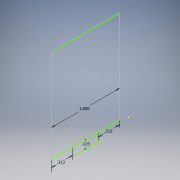
# Autodesk Inventor part: Part16
Saved by Autodesk Inventor 2018 (Build 220112000, 112)
## iProperties
Created: 2018-05-23
Part Number: Part16
Material: Generic
Document SubType Name: Modeling
Designer: lenovo
Density: 1 g/cm^3
Appearance: Default
Author: lenovo
Autodesk Inventor part; units mm, degrees
ref_plane "YZ Plane" through (0, 0, 0) normal (1, 0, 0) x (0, 1, 0)
ref_plane "XZ Plane" through (0, 0, 0) normal (0, 1, 0) x (-1, 0, 0)
ref_plane "XY Plane" through (0, 0, 0) normal (0, 0, 1) x (1, 0, 0)
sketch "Sketch1" plane through (0, 0, 0) normal (1, 0, 0) x (0, 1, 0)
  line L0 (35.589, 28.7672) -> (-47.596, 28.7672)
  line L1 (-47.596, 28.7672) -> (-47.596, 3.3672)
  line L2 (-47.596, 3.3672) -> (35.589, 3.3672)
  line L3 (35.589, 3.3672) -> (35.589, 28.7672)
  line L4 (-47.596, 20.8297) -> (-50.771, 20.8297)
  line L5 (-50.771, 20.8297) -> (-50.771, 11.3047)
  line L6 (-50.771, 11.3047) -> (-47.596, 11.3047)
  line L7 (-47.596, 11.3047) -> (-47.596, 20.8297)
  line L8 (-39.6585, 28.7672) -> (-30.1335, 28.7672)
  line L9 (-30.1335, 28.7672) -> (-30.1335, 25.5922)
  line L10 (-30.1335, 25.5922) -> (-39.6585, 25.5922)
  line L11 (-39.6585, 25.5922) -> (-39.6585, 28.7672)
  line L12 (-22.196, 20.8297) -> (-25.371, 20.8297)
  line L13 (-25.371, 20.8297) -> (-25.371, 11.3047)
  line L14 (-25.371, 11.3047) -> (-22.196, 11.3047)
  line L15 (-22.196, 11.3047) -> (-22.196, 20.8297)
  line L16 (-22.196, 3.3672) -> (-30.1335, 3.3672)
  line L17 (-30.1335, 3.3672) -> (-30.1335, 6.5422)
  line L18 (-30.1335, 6.5422) -> (-22.196, 6.5422)
  line L19 (-22.196, 6.5422) -> (-22.196, 3.3672)
  line L20 (-47.596, 3.3672) -> (-39.6585, 3.3672)
  line L21 (-39.6585, 3.3672) -> (-39.6585, 6.5422)
  line L22 (-39.6585, 6.5422) -> (-47.596, 6.5422)
  line L23 (-47.596, 6.5422) -> (-47.596, 3.3672)
  line L24 (35.589, 28.7672) -> (32.414, 28.7672)
  line L25 (32.414, 28.7672) -> (32.414, 20.8297)
  line L26 (32.414, 20.8297) -> (35.589, 20.8297)
  line L27 (35.589, 20.8297) -> (35.589, 28.7672)
  line L28 (35.589, 3.3672) -> (32.414, 3.3672)
  line L29 (32.414, 3.3672) -> (32.414, 11.3047)
  line L30 (32.414, 11.3047) -> (35.589, 11.3047)
  line L31 (35.589, 11.3047) -> (35.589, 3.3672)
  line L32 (27.6515, 3.3672) -> (18.1265, 3.3672)
  line L33 (18.1265, 3.3672) -> (18.1265, 6.5422)
  line L34 (18.1265, 6.5422) -> (27.6515, 6.5422)
  line L35 (27.6515, 6.5422) -> (27.6515, 3.3672)
  line L36 (27.6515, 28.7672) -> (18.1265, 28.7672)
  line L37 (18.1265, 28.7672) -> (18.1265, 25.5922)
  line L38 (18.1265, 25.5922) -> (27.6515, 25.5922)
  line L39 (27.6515, 25.5922) -> (27.6515, 28.7672)
  line L40 (13.364, 28.7672) -> (10.189, 28.7672)
  line L41 (10.189, 28.7672) -> (10.189, 20.8297)
  line L42 (10.189, 20.8297) -> (13.364, 20.8297)
  line L43 (13.364, 20.8297) -> (13.364, 28.7672)
  line L44 (13.364, 3.3672) -> (10.189, 3.3672)
  line L45 (10.189, 3.3672) -> (10.189, 11.3047)
  line L46 (10.189, 11.3047) -> (13.364, 11.3047)
  line L47 (13.364, 11.3047) -> (13.364, 3.3672)
  point P0 (0, 0)
  dimension "d0" = 25.4
  dimension "d1" = 3.175
  dimension "d2" = 7.9375
  dimension "d3" = 7.9375
  dimension "d4" = 83.185
  dimension "d5" = 3.175
  dimension "d6" = 9.525
  dimension "d7" = 7.9375
  dimension "d8" = 25.4
  dimension "d9" = 3.175
  dimension "d10" = 3.175
  dimension "d11" = 7.9375
  dimension "d12" = 3.175
  dimension "d13" = 7.9375
  dimension "d14" = 9.525
  dimension "d15" = 3.175
  dimension "d16" = 25.4
  constraints: 96 end point, 24 parallel, 12 horizontal, 12 perpendicular, 7 point on line, 1 collinear
  measures "d0" distance between parallel lines of L2 L0
  measures "d1" distance between parallel lines of L1 L5
  measures "d2" distance between parallel lines of L2 L6
  measures "d3" distance between parallel lines of L0 L4
  measures "d4" distance between parallel lines of L1 L3
  measures "d5" distance between parallel lines of L0 L10
  measures "d6" distance between parallel lines of L9 L11
  measures "d7" distance between parallel lines of L1 L11
  measures "d8" distance between parallel lines of L1 L15
  measures "d9" distance between parallel lines of L15 L13
  measures "d10" distance between parallel lines of L2 L18
  measures "d11" distance between parallel lines of L19 L17
  measures "d12" distance between parallel lines of L3 L25
  measures "d13" distance between parallel lines of L35 L3
  measures "d14" distance between parallel lines of L33 L35
  measures "d15" distance between parallel lines of L43 L41
  measures "d16" distance between parallel lines of L3 L41
extrude "Extrusion1" add sketch "Sketch1" along normal blind 3.175 contours L25 L26 L3 L30 L29 L2 L35 L34 L33 L47 L46 L45 L19 L18 L17 L21 L22 L1 L0 L11 L10 L9 L41 L42 L43 L37 L38 L39 | L1 L6 L5 L4
body "Solid1"
